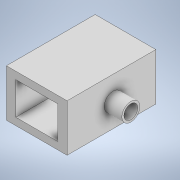
# Autodesk Inventor part: Part4
Saved by Autodesk Inventor 2020.3 (Build 243373000, 373)
## iProperties
Created: 2021-01-23
Part Number: Part4
Material: Generic
Document SubType Name: Modeling
Designer: Yu Jinyu
Density: 1 g/cm^3
Appearance: Default
Author: Yu Jinyu
Autodesk Inventor part; units mm, degrees
ref_plane "YZ Plane" through (0, 0, 0) normal (1, 0, 0) x (0, 1, 0)
ref_plane "XZ Plane" through (0, 0, 0) normal (0, 1, 0) x (-1, 0, 0)
ref_plane "XY Plane" through (0, 0, 0) normal (0, 0, 1) x (1, 0, 0)
sketch "Sketch1" plane through (0, 0, 0) normal (0, 0, 1) x (1, 0, 0)
  line L0 (-3.4184, -2.6565) -> (3.4184, -2.6565)
  line L1 (3.4184, -2.6565) -> (3.4184, 2.6565)
  line L2 (3.4184, 2.6565) -> (-3.4184, 2.6565)
  line L3 (-3.4184, 2.6565) -> (-3.4184, -2.6565)
  line L4 (-3.4184, -2.6565) -> (3.4184, 2.6565) construction
  line L5 (3.4184, -2.6565) -> (-3.4184, 2.6565) construction
  line L6 (-2.3603, -1.8342) -> (2.3603, -1.8342)
  line L7 (2.3603, -1.8342) -> (2.3603, 1.8342)
  line L8 (2.3603, 1.8342) -> (-2.3603, 1.8342)
  line L9 (-2.3603, 1.8342) -> (-2.3603, -1.8342)
  line L10 (-2.3603, -1.8342) -> (2.3603, 1.8342) construction
  line L11 (2.3603, -1.8342) -> (-2.3603, 1.8342) construction
  point P0 (0, 0)
  constraints: 24 end point, 4 midpoint, 4 parallel, 2 horizontal, 2 perpendicular, 1 point on line
extrude "Extrusion1" add sketch "Sketch1" along normal blind 10
sketch "Sketch2" plane through (3.4184, -2.6565, 0) normal (1, 0, 0) x (0, 0, -1)
  circle A0 centre (-4.8161, 2.6565) radius 1.0093
  circle A1 centre (-4.8161, 2.6565) radius 0.782
  point P0 (0, 2.6565)
  constraints: 2 centre point, 1 coincident
extrude "Extrusion2" add sketch "Sketch2" along normal blind 2
body "Solid1"
